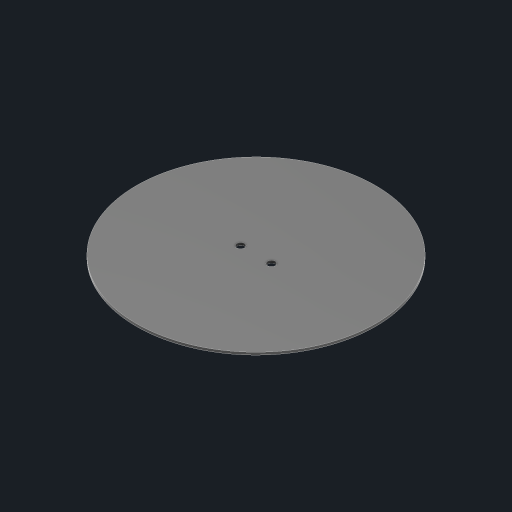
# Autodesk Inventor part: OUTK_008_Plunger
Saved by Autodesk Inventor 2024.2 (Build 282272000, 272)
## iProperties
Created: 2024-11-27
Part Number: OUTK_008_Plunger
Material: Acetal Resin, Black
Document SubType Name: Modeling
Designer: Bryan
Density: 1.425 g/cm^3
Appearance: Smooth - Black
Author: Bryan
Autodesk Inventor part; units mm, degrees
ref_plane "YZ Plane" through (0, 0, 0) normal (1, 0, 0) x (0, 1, 0)
ref_plane "XZ Plane" through (0, 0, 0) normal (0, 1, 0) x (-1, 0, 0)
ref_plane "XY Plane" through (0, 0, 0) normal (0, 0, 1) x (1, 0, 0)
sketch "Sketch1" plane through (0, 0, 0) normal (0, 1, 0) x (-1, 0, 0)
  circle A0 centre (0, 0) radius 76.2
  dimension "d0" = 152.4
  constraints: 1 centre point, 1 coincident
  measures "d0" diameter of A0
extrude "Extrusion1" add sketch "Sketch1" along normal blind 1.5875
sketch "Sketch2" plane through (0, 1.5875, 0) normal (0, 1, 0) x (1, 0, 0)
  circle A0 centre (-9.8414, 0) radius 2.4892
  circle A1 centre (9.8414, 0) radius 2.4892
  line L0 (0, 0) -> (0, 2.4892) construction
  dimension "d3" = 4.9784
  dimension "d4" = 4.9784
  dimension "d5" = 19.6829
  constraints: 2 centre point, 2 end point, 1 horizontal alignment, 1 symmetric about line, 1 vertical
  measures "d3" diameter of A0
  measures "d4" diameter of A1
  measures "d5" distance of A1.centre A0.centre
extrude "Extrusion2" cut sketch "Sketch2" against normal through all
body "Solid1"
